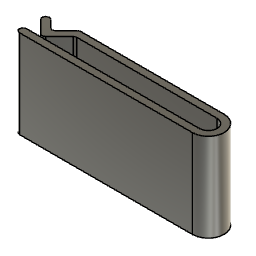
Desktop Cable Management Clip v1 (Autodesk Fusion 360 design; units mm, degrees)
Autodesk Fusion 360 part; units mm, degrees
sketch "Sketch1" plane through (0, 0, 0) normal (0, 0, 1) x (1, 0, 0)
  line L0 (0, 0) -> (50, 0)
  arc A0 (50, 0) -> (50, 5) centre (50, 2.5) ccw
  line L1 (50, 5) -> (9.8, 5)
  line L2 (9.8, 5) -> (4.9, 0.1)
  line L3 (4.9, 0.1) -> (0, 5)
  line L4 (0, -2) -> (50, -2)
  arc A1 (50, -2) -> (50, 7) centre (50, 2.5) ccw
  line L5 (50, 7) -> (8.9716, 7)
  line L6 (8.9716, 7) -> (4.9, 2.9284)
  line L7 (4.9, 2.9284) -> (1.4142, 6.4142)
  line L8 (0, -2) -> (0, 0)
  line L9 (0, 5) -> (1.4142, 6.4142)
  dimension "d4" = 135
  dimension "d5" = 50
  dimension "d6" = 5
  dimension "d8" = 0.1
  constraint coincident L0.start L8.end
  constraint horizontal L0
  constraint tangent L0 A0
  constraint tangent A0 L1
  constraint parallel L0 L1
  constraint perpendicular L2 L3
  constraint coincident L1 L3.end
  constraint vertical L0.start L3.end
  constraint perpendicular L0 L8
  constraint concentric A0 A1
  constraint tangent L4 A1
  constraint tangent A1 L5
  constraint coincident L2.end L3.start
  constraint perpendicular L7 L9
  measures "d4" angle of L1 L2
  measures "d5" distance of L0.start L0.end
  measures "d6" distance of L0 L1
  measures "d8" distance of L0 L2.end
extrude "Extrude1" add sketch "Sketch1" along normal blind 25
fillet "Fillet1" radius 1 8 edges at (4.9, 2.9284, 12.5) (4.9, 0.1, 12.5) (9.8, 5, 12.5) (8.9716, 7, 12.5) (1.4142, 6.4142, 12.5) (0, 5, 12.5) (0, -2, 12.5) (0, 0, 12.5)
